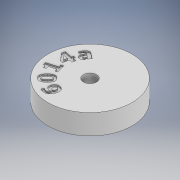
# Autodesk Inventor part: Extruder_Hot_End_Spacer_LM6014
Saved by Autodesk Inventor 2020.2 (Build 242310000, 310)
## iProperties
Created: 2020-04-13
Part Number: Extruder_Hot_End_Spacer_LM6014
Material: Generic
Document SubType Name: Modeling
Designer: rah75
Density: 1 g/cm^3
Appearance: Default
Author: rah75
Autodesk Inventor part; units mm, degrees
ref_plane "YZ Plane" through (0, 0, 0) normal (1, 0, 0) x (0, 1, 0)
ref_plane "XZ Plane" through (0, 0, 0) normal (0, 1, 0) x (-1, 0, 0)
ref_plane "XY Plane" through (0, 0, 0) normal (0, 0, 1) x (1, 0, 0)
sketch "Sketch1" plane through (0, 0, 0) normal (0, 1, 0) x (-1, 0, 0)
  circle A0 centre (0, 0) radius 8
  circle A1 centre (0, 0) radius 1.25
  dimension "d0" = 16
  dimension "d1" = 2.5
  constraints: 2 centre point, 2 coincident
  measures "d0" diameter of A0
  measures "d1" diameter of A1
extrude "Extrusion1" add sketch "Sketch1" along normal blind 3.85
sketch "Sketch2" plane through (0, 3.85, 0) normal (0, 1, 0) x (1, 0, 0)
  arc A0 (-0.3119, 4.4892) -> (-0.3119, -4.4892) centre (0, 0) ccw
  spline S0 degree 2 poles (-2.5946, -4.8001) (-2.4715, -4.418) (-1.8291, -4.0822) (-1.4059, -4.2186) knots 0 0 0 1 2 2 2
  spline S1 degree 2 poles (-1.4059, -4.2186) (-1.1944, -4.2868) (-0.9024, -4.5149) (-0.8253, -4.6717) knots 0 0 0 1 2 2 2
  spline S2 degree 2 poles (-0.8253, -4.6717) (-0.733, -4.855) (-0.7281, -5.3431) (-0.8273, -5.6507) knots 0 0 0 1 2 2 2
  spline S3 degree 2 poles (-0.8273, -5.6507) (-0.9295, -5.9681) (-1.2258, -6.4176) (-1.4418, -6.5578) knots 0 0 0 1 2 2 2
  spline S4 degree 2 poles (-1.4418, -6.5578) (-1.6468, -6.6907) (-2.1905, -6.7404) (-2.5177, -6.6349) knots 0 0 0 1 2 2 2
  spline S5 degree 2 poles (-2.5177, -6.6349) (-2.6372, -6.5964) (-2.8661, -6.4881) (-2.906, -6.4644) knots 0 0 0 1 2 2 2
  line L0 (-2.906, -6.4644) -> (-2.7532, -5.9903)
  line L1 (-2.7532, -5.9903) -> (-2.7101, -6.0041)
  spline S6 degree 2 poles (-2.7101, -6.0041) (-2.674, -6.0396) (-2.4951, -6.1556) (-2.3697, -6.196) knots 0 0 0 1 2 2 2
  spline S7 degree 2 poles (-2.3697, -6.196) (-2.0857, -6.2876) (-1.6795, -6.0876) (-1.5526, -5.8214) knots 0 0 0 1 2 2 2
  spline S8 degree 2 poles (-1.5526, -5.8214) (-1.6968, -5.8593) (-1.9707, -5.8705) (-2.1255, -5.8206) knots 0 0 0 1 2 2 2
  spline S9 degree 2 poles (-2.1255, -5.8206) (-2.2567, -5.7783) (-2.4632, -5.6339) (-2.5299, -5.5389) knots 0 0 0 1 2 2 2
  spline S10 degree 2 poles (-2.5299, -5.5389) (-2.6244, -5.4025) (-2.6729, -5.043) (-2.5946, -4.8001) knots 0 0 0 1 2 2 2
  spline S11 degree 2 poles (-1.7699, -4.6636) (-1.8359, -4.7072) (-1.931, -4.8279) (-1.9758, -4.967) knots 0 0 0 1 2 2 2
  spline S12 degree 2 poles (-1.9758, -4.967) (-2.0137, -5.0846) (-2.0042, -5.2563) (-1.9658, -5.3184) knots 0 0 0 1 2 2 2
  spline S13 degree 2 poles (-1.9658, -5.3184) (-1.9261, -5.3831) (-1.8017, -5.46) (-1.7253, -5.4846) knots 0 0 0 1 2 2 2
  spline S14 degree 2 poles (-1.7253, -5.4846) (-1.6606, -5.5054) (-1.5167, -5.5151) (-1.4503, -5.5105) knots 0 0 0 1 2 2 2
  spline S15 degree 2 poles (-1.4503, -5.5105) (-1.4453, -5.4948) (-1.4173, -5.4216) (-1.399, -5.3648) knots 0 0 0 1 2 2 2
  spline S16 degree 2 poles (-1.399, -5.3648) (-1.3315, -5.1552) (-1.3225, -4.8791) (-1.3585, -4.7961) knots 0 0 0 1 2 2 2
  spline S17 degree 2 poles (-1.3585, -4.7961) (-1.3826, -4.73) (-1.4778, -4.6496) (-1.5366, -4.6306) knots 0 0 0 1 2 2 2
  spline S18 degree 2 poles (-1.5366, -4.6306) (-1.5855, -4.6149) (-1.715, -4.6272) (-1.7699, -4.6636) knots 0 0 0 1 2 2 2
  spline S19 degree 2 poles (-4.8094, -3.3348) (-4.5739, -3.1045) (-4.1473, -2.8342) (-3.9461, -2.8015) knots 0 0 0 1 2 2 2
  spline S20 degree 2 poles (-3.9461, -2.8015) (-3.7478, -2.7687) (-3.3666, -2.9171) (-3.1795, -3.1083) knots 0 0 0 1 2 2 2
  spline S21 degree 2 poles (-3.1795, -3.1083) (-2.991, -3.3011) (-2.8526, -3.684) (-2.8912, -3.8859) knots 0 0 0 1 2 2 2
  spline S22 degree 2 poles (-2.8912, -3.8859) (-2.9284, -4.0864) (-3.2052, -4.5039) (-3.4406, -4.7342) knots 0 0 0 1 2 2 2
  spline S23 degree 2 poles (-3.4406, -4.7342) (-3.682, -4.9703) (-4.0968, -5.2291) (-4.3038, -5.2647) knots 0 0 0 1 2 2 2
  spline S24 degree 2 poles (-4.3038, -5.2647) (-4.508, -5.2973) (-4.8891, -5.1432) (-5.0704, -4.9578) knots 0 0 0 1 2 2 2
  spline S25 degree 2 poles (-5.0704, -4.9578) (-5.2618, -4.7621) (-5.3944, -4.3792) (-5.3543, -4.1759) knots 0 0 0 1 2 2 2
  spline S26 degree 2 poles (-5.3543, -4.1759) (-5.3157, -3.9769) (-5.0374, -3.5579) (-4.8094, -3.3348) knots 0 0 0 1 2 2 2
  spline S27 degree 2 poles (-4.3617, -3.7925) (-4.6987, -4.122) (-4.863, -4.4987) (-4.7349, -4.6296) knots 0 0 0 1 2 2 2
  spline S28 degree 2 poles (-4.7349, -4.6296) (-4.6068, -4.7606) (-4.2252, -4.6062) (-3.8868, -4.2751) knots 0 0 0 1 2 2 2
  spline S29 degree 2 poles (-3.8868, -4.2751) (-3.5542, -3.9499) (-3.3869, -3.5675) (-3.515, -3.4365) knots 0 0 0 1 2 2 2
  spline S30 degree 2 poles (-3.515, -3.4365) (-3.6417, -3.307) (-4.0277, -3.4657) (-4.3617, -3.7925) knots 0 0 0 1 2 2 2
  line L2 (-4.5692, -0.4239) -> (-4.0902, -2.0316)
  line L3 (-4.0902, -2.0316) -> (-4.5143, -2.1579)
  line L4 (-4.5143, -2.1579) -> (-4.6671, -1.6451)
  line L5 (-4.6671, -1.6451) -> (-5.9553, -2.0289)
  line L6 (-5.9553, -2.0289) -> (-5.8025, -2.5417)
  line L7 (-5.8025, -2.5417) -> (-6.199, -2.6599)
  spline S31 degree 2 poles (-6.199, -2.6599) (-6.2325, -2.5474) (-6.3285, -2.3333) (-6.38, -2.2757) knots 0 0 0 1 2 2 2
  spline S32 degree 2 poles (-6.38, -2.2757) (-6.4424, -2.2105) (-6.6004, -2.1631) (-6.7014, -2.1846) knots 0 0 0 1 2 2 2
  line L8 (-6.7014, -2.1846) -> (-6.8601, -1.652)
  line L9 (-6.8601, -1.652) -> (-4.844, -1.0513)
  line L10 (-4.844, -1.0513) -> (-4.9933, -0.5502)
  line L11 (-4.9933, -0.5502) -> (-4.5692, -0.4239)
  line L12 (-4.7939, 2.0104) -> (-4.8606, 1.6732)
  line L13 (-4.8606, 1.6732) -> (-4.273, 1.557)
  line L14 (-4.273, 1.557) -> (-4.3923, 0.9533)
  line L15 (-4.3923, 0.9533) -> (-4.9799, 1.0694)
  line L16 (-4.9799, 1.0694) -> (-5.1971, -0.029)
  line L17 (-5.1971, -0.029) -> (-5.6615, 0.0628)
  line L18 (-5.6615, 0.0628) -> (-6.8942, 1.4269)
  line L19 (-6.8942, 1.4269) -> (-6.7708, 2.0508)
  line L20 (-6.7708, 2.0508) -> (-5.3089, 1.7618)
  line L21 (-5.3089, 1.7618) -> (-5.2422, 2.099)
  line L22 (-5.2422, 2.099) -> (-4.7939, 2.0104)
  line L23 (-5.4282, 1.1581) -> (-6.2763, 1.3257)
  line L24 (-6.2763, 1.3257) -> (-5.5532, 0.526)
  line L25 (-5.5532, 0.526) -> (-5.4282, 1.1581)
  spline S33 degree 2 poles (-3.5515, 3.0934) (-3.5492, 3.0131) (-3.5442, 2.8861) (-3.5627, 2.796) knots 0 0 0 1 2 2 2
  spline S34 degree 2 poles (-3.5627, 2.796) (-3.5815, 2.7087) (-3.6432, 2.5635) (-3.7272, 2.4566) knots 0 0 0 1 2 2 2
  spline S35 degree 2 poles (-3.7272, 2.4566) (-3.8848, 2.2559) (-4.3608, 2.2032) (-4.5647, 2.3634) knots 0 0 0 1 2 2 2
  spline S36 degree 2 poles (-4.5647, 2.3634) (-4.7315, 2.4943) (-4.8331, 2.7914) (-4.7938, 2.9647) knots 0 0 0 1 2 2 2
  spline S37 degree 2 poles (-4.7938, 2.9647) (-4.7549, 3.1409) (-4.525, 3.5336) (-4.3777, 3.7477) knots 0 0 0 1 2 2 2
  line L26 (-4.3777, 3.7477) -> (-4.3858, 3.754)
  spline S38 degree 2 poles (-4.3858, 3.754) (-4.5105, 3.8519) (-4.7509, 3.7424) (-4.8959, 3.5579) knots 0 0 0 1 2 2 2
  spline S39 degree 2 poles (-4.8959, 3.5579) (-4.9607, 3.4754) (-5.0763, 3.2049) (-5.112, 3.0628) knots 0 0 0 1 2 2 2
  line L27 (-5.112, 3.0628) -> (-5.1438, 3.0224)
  line L28 (-5.1438, 3.0224) -> (-5.508, 3.3085)
  spline S40 degree 2 poles (-5.508, 3.3085) (-5.4727, 3.3933) (-5.2836, 3.7473) (-5.159, 3.906) knots 0 0 0 1 2 2 2
  spline S41 degree 2 poles (-5.159, 3.906) (-4.8539, 4.2944) (-4.3151, 4.4471) (-4.0497, 4.2386) knots 0 0 0 1 2 2 2
  line L29 (-4.0497, 4.2386) -> (-3.0251, 3.4337)
  line L30 (-3.0251, 3.4337) -> (-3.3913, 2.9676)
  line L31 (-3.3913, 2.9676) -> (-3.5515, 3.0934)
  line L32 (-3.7846, 3.2765) -> (-4.097, 3.5219)
  spline S42 degree 2 poles (-4.097, 3.5219) (-4.1798, 3.3932) (-4.2777, 3.232) (-4.3077, 3.1404) knots 0 0 0 1 2 2 2
  spline S43 degree 2 poles (-4.3077, 3.1404) (-4.3363, 3.0607) (-4.3022, 2.9241) (-4.231, 2.8681) knots 0 0 0 1 2 2 2
  spline S44 degree 2 poles (-4.231, 2.8681) (-4.1258, 2.7855) (-3.9562, 2.8381) (-3.8685, 2.9498) knots 0 0 0 1 2 2 2
  spline S45 degree 2 poles (-3.8685, 2.9498) (-3.8202, 3.0113) (-3.7751, 3.1853) (-3.7846, 3.2765) knots 0 0 0 1 2 2 2
  dimension "d4" = 4.5
  constraints: 2 point on circle, 1 centre point, 1 coincident, 1 vertical alignment, 1 other
  measures "d4" radius of A0
emboss "Emboss1" sketch "Sketch2" operation cut depth 0.25 direction (0, -1, 0)
body "Solid1"
